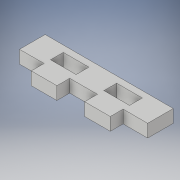
# Autodesk Inventor part: thumper-bumper-sidewall2-v3
Saved by Autodesk Inventor 2017 (Build 210142000, 142)
## iProperties
Created: 2017-02-22
Part Number: thumper-bumper-sidewall2-v3
Material: Generic
Document SubType Name: Modeling
Designer: John
Density: 1 g/cm^3
Appearance: Default
Author: John
Autodesk Inventor part; units mm, degrees
ref_plane "YZ Plane" through (0, 0, 0) normal (1, 0, 0) x (0, 1, 0)
ref_plane "XZ Plane" through (0, 0, 0) normal (0, 1, 0) x (-1, 0, 0)
ref_plane "XY Plane" through (0, 0, 0) normal (0, 0, 1) x (1, 0, 0)
sketch "Sketch1" plane through (0, 0, 0) normal (0, 1, 0) x (-1, 0, 0)
  line L0 (27.5, 50.0814) -> (27.5, 62.0814)
  line L1 (-32.5, 62.0814) -> (-32.5, 50.0814)
  line L2 (-32.5, 50.0814) -> (-2.5, 50.0814)
  line L3 (-2.5, 50.0814) -> (-2.5, 62.0814) construction
  line L4 (-32.5, 56.0814) -> (-2.5, 56.0814) construction
  line L5 (-32.5, 62.0814) -> (27.5, 62.0814)
  line L6 (-21, 62.0814) -> (-9, 62.0814)
  line L7 (-9, 62.0814) -> (-9, 68.0814)
  line L8 (-9, 68.0814) -> (-21, 68.0814)
  line L9 (-21, 68.0814) -> (-21, 62.0814)
  line L10 (16, 62.0814) -> (4, 62.0814)
  line L11 (4, 62.0814) -> (4, 68.0814)
  line L12 (4, 68.0814) -> (16, 68.0814)
  line L13 (16, 68.0814) -> (16, 62.0814)
  line L14 (-2.5, 56.0814) -> (27.5, 56.0814) construction
  line L15 (-2.5, 50.0814) -> (27.5, 50.0814)
  line L16 (-9, 59.0814) -> (-21, 59.0814)
  line L17 (-21, 59.0814) -> (-21, 53.0814)
  line L18 (-21, 53.0814) -> (-9, 53.0814)
  line L19 (-9, 53.0814) -> (-9, 59.0814)
  line L20 (-9, 59.0814) -> (-21, 53.0814) construction
  line L21 (-21, 59.0814) -> (-9, 53.0814) construction
  line L22 (4, 59.0814) -> (16, 59.0814)
  line L23 (16, 59.0814) -> (16, 53.0814)
  line L24 (16, 53.0814) -> (4, 53.0814)
  line L25 (4, 53.0814) -> (4, 59.0814)
  line L26 (4, 59.0814) -> (16, 53.0814) construction
  line L27 (16, 59.0814) -> (4, 53.0814) construction
  point P0 (-15, 56.0814)
  point P1 (10, 56.0814)
  dimension "d0" = 60
  dimension "d1" = 12
  dimension "d18" = 12
  dimension "d19" = 6
  dimension "d20" = 18.5
  dimension "d21" = 12
  dimension "d22" = 6
  dimension "d23" = 3
  constraints: 56 end point, 9 symmetric about line, 7 midpoint, 7 parallel, 5 horizontal, 2 equal length, 2 perpendicular, 1 collinear, 1 point on line, 1 vertical
  measures "d0" distance of L1.start L0.end
  measures "d1" distance of L0.end L0.start
  measures "d18" distance of L8.end L7.end
  measures "d19" distance of L7.end L6.end
  measures "d20" distance between parallel lines of L3 L9
  measures "d21" distance of L18.end L17.end
  measures "d22" distance of L17.end L16.end
  measures "d23" distance between parallel lines of L5 L16
extrude "Extrusion1" add sketch "Sketch1" along normal blind 6
sketch "Sketch3" plane through (0, 0, 0) normal (0, 1, 0) x (-1, 0, 0)
  line L0 (4, 62.0814) -> (-9, 62.0814) construction
  line L1 (-2.5, 62.0814) -> (-2.5, 50.0814) construction
  line L2 (-32.5, 50.0814) -> (27.5, 50.0814) construction
  line L3 (8.5, 50.0814) -> (2.5, 50.0814)
  line L4 (2.5, 50.0814) -> (2.5, 44.0814)
  line L5 (2.5, 44.0814) -> (8.5, 44.0814)
  line L6 (8.5, 44.0814) -> (8.5, 50.0814)
  line L7 (8.5, -0.9186) -> (2.5, -0.9186)
  line L8 (2.5, -0.9186) -> (2.5, -6.9186)
  line L9 (2.5, -6.9186) -> (8.5, -6.9186)
  line L10 (8.5, -6.9186) -> (8.5, -0.9186)
  line L11 (8.5, 35.0814) -> (-9.5, 35.0814)
  line L12 (-9.5, 35.0814) -> (-9.5, 23.0814)
  line L13 (-9.5, 13.0814) -> (8.5, 13.0814)
  line L14 (8.5, 13.0814) -> (8.5, 23.0814)
  line L15 (-13, 35.0814) -> (12, 35.0814)
  line L16 (8.5, 23.0814) -> (-9.5, 23.0814)
  line L17 (1.5, 35.0814) -> (-5.5, 35.0814)
  line L18 (-5.5, 35.0814) -> (-5.5, 40.0814)
  line L19 (-5.5, 40.0814) -> (1.5, 40.0814)
  line L20 (1.5, 40.0814) -> (1.5, 35.0814)
  line L21 (-9.5, 23.0814) -> (-9.5, 13.0814)
  line L22 (8.5, 23.0814) -> (8.5, 35.0814)
  point P0 (0, 0)
  dimension "d37" = 6
  dimension "d38" = 6
  dimension "d39" = 6
  dimension "d43" = 12
  dimension "d44" = 45
  dimension "d45" = 5
  dimension "d46" = 18
  dimension "d47" = 22
  dimension "d53" = 9
  dimension "d58" = 7
  dimension "d59" = 5
  dimension "d60" = 1
  constraints: 42 end point, 12 parallel, 5 collinear, 5 horizontal, 5 perpendicular, 2 midpoint, 1 point on line
  measures "d37" distance of L5.end L4.end
  measures "d38" distance of L4.end L3.end
  measures "d39" distance of L8.end L7.end
  measures "d43" distance between parallel lines of L0 L3
  measures "d44" distance between parallel lines of L7 L5
  measures "d45" distance between parallel lines of L1 L4
  measures "d46" distance of L13.end L13.start
  measures "d47" distance of L13.start L11.end
  measures "d53" distance between parallel lines of L5 L11
  measures "d58" distance of L18.end L19.end
  measures "d59" distance of L17.end L18.end
  measures "d60" distance between parallel lines of L20 L4
extrude "Extrusion3" cut sketch "Sketch3" along normal through all
body "Solid1"
